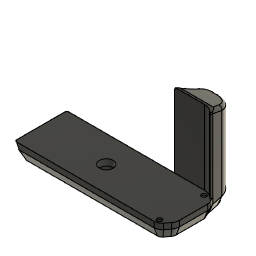
Fujifilm_XE4_Grip (Autodesk Fusion 360 design; units mm, degrees)
Autodesk Fusion 360 part; units mm, degrees
note: some values were not read from the file. Chosen so that the rebuilt part matches the saved one: which pieces of a blend or face edit are solid. Set by a fixed rule: which sketch regions a step uses.
sketch "Boceto1" plane through (0, 0, 0) normal (0, 0, 1) x (1, 0, 0)
  line L0 (-61.186123, 0) -> (71.866078, 0)
  line L1 (-61.186123, 16.5) -> (58.439032, 16.5)
  line L2 (-61.186123, -15.8) -> (59.434444, -15.8)
  line L3 (0, 28.622619) -> (0, -27.140205)
  line L4 (66.8, 10.132205) -> (66.8, -7.372166)
  line L5 (62.761803, 15.128919) -> (63.868179, 14.348585)
  arc A0 (62.761803, 15.128919) -> (58.439032, 16.5) centre (58.439032, 9) ccw
  line L6 (64.040509, 14.215674) -> (65.452845, 13.026924)
  arc A1 (66.8, 10.132205) -> (65.452845, 13.026924) centre (63.016387, 10.132205) ccw
  arc A2 (64.040509, 14.215674) -> (63.868179, 14.348585) centre (62.398436, 12.264752) ccw
  circle A3 centre (52.520822, 19.704936) radius 11.20941
  line L7 (52.520822, 30.914346) -> (49.214141, 30.914346)
  arc A4 (39.279231, 16.5) -> (43.791824, 26.33548) centre (23.188368, 29.835558) ccw
  arc A5 (49.214141, 30.914346) -> (43.791824, 26.33548) centre (49.214141, 25.414346) ccw
  line L8 (41.763113, 20.257885) -> (39.82544, 16.5)
  line L9 (65.452845, 13.026924) -> (63.472116, 22.096594)
  circle A6 centre (62.754834, 14.530444) radius 2.315092
  circle A7 centre (14, 0) radius 4.25
  circle A8 centre (14, 0) radius 6.75
  line L10 (-27, 16.5) -> (-27, -15.8)
  line L11 (35.876287, -15.8) -> (35.876287, -16.8)
  line L12 (35.876287, -16.8) -> (57.161819, -16.8)
  line L13 (57.161819, -16.8) -> (57.161819, -15.8)
  circle A9 centre (60.249431, -13.250185) radius 1.5
  circle A10 centre (60.988338, 13.604964) radius 1.5
  line L14 (63.404093, -13.840047) -> (65.563579, -11.020223)
  arc A11 (59.434444, -15.8) -> (63.404093, -13.840047) centre (59.434444, -10.8) ccw
  arc A12 (65.563579, -11.020223) -> (66.8, -7.372166) centre (60.8, -7.372166) ccw
  dimension "d4" = 7.5
  dimension "d6" = 2.55
  dimension "d7" = 5.5
  dimension "d8" = 8.5
  dimension "d9" = 13.5
  dimension "d14" = 1
  dimension "d15" = 3
  dimension "d16" = 3
  dimension "d17" = 5
  dimension "d18" = 6
  dimension "d41" = 16.5
  dimension "d42" = 15.8
  dimension "d43" = 66.8
  dimension "d44" = 14
  constraint horizontal L0
  constraint perpendicular L2 L3
  constraint parallel L0 L1
  constraint tangent L1 A0
  constraint tangent L5 A0
  constraint parallel L3 L4
  constraint tangent L6 A1
  constraint tangent L4 A1
  constraint tangent L5 A2
  constraint tangent L6 A2
  constraint tangent A3 L7
  constraint horizontal L7
  constraint tangent L7 A5
  constraint tangent A4 A5
  constraint tangent A4 L8
  constraint tangent A3 L9
  constraint tangent L9 A6
  constraint concentric A7 A8
  constraint parallel L0 L2
  constraint perpendicular L2 L11
  constraint perpendicular L11 L12
  constraint perpendicular L2 L13
  constraint tangent L2 A11
  constraint tangent L14 A11
  constraint tangent L14 A12
  constraint tangent L4 A12
  constraint coincident origin L0
  constraint horizontal origin A7.centre
  constraint coincident L1 L10.start
  constraint coincident L2 L10.end
  measures "d4" radius of A0
  measures "d6" radius of A2
  measures "d7" radius of A5
  measures "d8" diameter of A7
  measures "d9" diameter of A8
  measures "d15" diameter of A9
  measures "d16" diameter of A10
  measures "d17" radius of A11
  measures "d18" radius of A12
  measures "d41" distance of L0 L1
  measures "d42" distance of L0 L2
  measures "d43" distance of origin L4
  measures "d44" horizontal distance of origin A7.centre
extrude "Extruir1" add sketch "Boceto1" against normal blind 9 contours L0 A7 A8 | L0 A7 A8 | L0 L1 L3 L4 L6 A1 A3 A6 A8 A10 | L0 L2 L3 L4 A8 L14 A11 A12 | L0 L2 L3 L10 | L0 L1 L3 L10 | L5 A0 L6 A2 A3 A6 A10 | L5 A0 L6 A2 A3 A6 | A3 L9 A6 | A3 A6 A10 | A3 A6 A10 | L1 A0 A3 A4 A5 L8 A6 | A0 A3 A6 | L1 A3 L8 | A3 A6 A10 | A3 A6 A10 | L1 A0 A3 A6 A10 | A3 L7 A5 | A0 A3 A6 A10 | A9 picked at (11.344649, 5.269892) picked at (8.108464, -0.335345) picked at (18.260416, 13.193588) picked at (41.142096, -5.266667) picked at (-18, -5.266667) picked at (-18, 11) picked at (63.509623, 13.402236) picked at (63.825041, 15.302467) picked at (63.810413, 17.600151) picked at (61.317784, 12.424239) picked at (62.039166, 13.392483) picked at (50.353547, 23.728105) picked at (62.520167, 15.99099) picked at (41.048535, 16.816247) picked at (61.414822, 14.237939) picked at (60.789556, 12.505385) picked at (58.292127, 13.195865) picked at (47.006875, 29.774605) picked at (61.192246, 15.569708) picked at (59.87732, -12.98462)
extrude "Extruir2" cut sketch "Boceto1" along normal blind -4 and the other way blind 9 contours L0 A7 A8 | L0 A7 A8 picked at (11.344649, 5.269892) picked at (8.108464, -0.335345)
extrude "Extruir3" add sketch "Boceto1" along normal blind 48 contours L5 A0 L6 A2 A3 A6 | A3 L9 A6 | L1 A0 A3 A4 A5 L8 A6 | A0 A3 A6 | L1 A3 L8 | A3 L7 A5 picked at (63.825041, 15.302467) picked at (63.810413, 17.600151) picked at (50.353547, 23.728105) picked at (62.520167, 15.99099) picked at (41.048535, 16.816247) picked at (47.006875, 29.774605)
sketch "Boceto2" plane through (0, 0, 0) normal (1, 0, 0) x (0, 1, 0)
  line L0 (0, 0) -> (0, 41.347667)
  line L1 (0, 41.347667) -> (34.217677, 41.347667)
  line L2 (31.646617, 41.347667) -> (6.75876, 49.907463)
  line L3 (6.75876, 49.907463) -> (34.217677, 49.907463)
  line L4 (34.217677, 49.907463) -> (34.217677, 41.347667)
  dimension "d45" = 41.347667
  constraint coincident L0.start origin
  constraint vertical L0
  constraint perpendicular L0 L1
  constraint parallel L1 L3
  constraint perpendicular L1 L4
extrude "Extruir4" cut sketch "Boceto2" along normal blind 110 contours L1 L2 L3 L4 picked at (24.207685, 47.054198)
fillet "Empalme1" radius 2 7 edges at (40.794276, 18.378943, 45.91088) (43.011767, 23.218473, 44.246398) (45.665636, 29.616502, 42.045894) (50.867481, 30.914346, 41.59952) (59.550822, 28.435914, 42.451939) (64.244366, 18.560495, 45.848438) (65.054866, 14.266815, 47.325183)
chamfer "Chaflán1" distance 4.2 distance2 9 1 edges at (-27, 0.35, -9) measured on face at (-15.583333, 0.233333, -9)
fillet "Empalme2" radius 9 1 edges at (64.846194, 13.537537, -4.5)
chamfer "Chaflán2" distance 2.2 distance2 5.5 14 edges at (8.51272, 16.5, -9) (43.011767, 23.218473, -9) (40.794276, 18.378943, -9) (18.317222, -15.8, -9) (61.648011, -15.283316, -9) (64.483836, -12.430135, -9) (66.482494, -9.298111, -9) (66.8, 1.38002, -9) (66.648742, 11.19132, -9) (65.47665, 13.571068, -9) (64.238004, 18.589627, -9) (59.550822, 28.435914, -9) (50.867481, 30.914346, -9) (45.665636, 29.616502, -9) measured on face at (-12.783893, 0.233333, -9) measured on face at (-12.783893, 0.233333, -9) measured on face at (-12.783893, 0.233333, -9) measured on face at (-12.783893, 0.233333, -9) measured on face at (-12.783893, 0.233333, -9) measured on face at (-12.783893, 0.233333, -9) measured on face at (-12.783893, 0.233333, -9) measured on face at (-12.783893, 0.233333, -9) measured on face at (-12.783893, 0.233333, -9) measured on face at (65.411059, 13.734607, -6) measured on face at (-12.783893, 0.233333, -9) measured on face at (-12.783893, 0.233333, -9) measured on face at (-12.783893, 0.233333, -9) measured on face at (-12.783893, 0.233333, -9)
chamfer "Chaflán3" distance 0.5 distance2 1 1 edges at (7.70679, -2.440904, -9) measured on face at (-12.783893, 0.233333, -9)
extrude "Extruir5" cut sketch "Boceto1" against normal blind 1 contours A3 A6 A10 | A3 A6 A10 | A3 A6 A10 | A3 A6 A10 | A9 picked at (61.317784, 12.424239) picked at (62.039166, 13.392483) picked at (61.414822, 14.237939) picked at (60.789556, 12.505385) picked at (59.87732, -12.98462)
fillet "Fillet3" radius 1 4 edges at (-24.083333, -14.7, -6.25) (-26.183333, -15.8, -1.75) (-26.183333, 16.5, -1.75) (-24.083333, 15.4, -6.25)
sketch "Trim" plane through (0, 0, 0) normal (0, 1, 0) x (1, 0, 0)
  line L0 (68.315111, -54.700248) -> (37.362685, -54.700248)
  line L1 (37.362685, -54.700248) -> (37.362685, -46.105812)
  line L2 (37.362685, -46.105812) -> (68.315111, -46.105812)
  line L3 (68.315111, -46.105812) -> (68.315111, -54.700248)
  constraint horizontal L0
  constraint vertical L1
  constraint horizontal L2
  constraint vertical L3
extrude "Extrude6" cut sketch "Trim" along normal blind 29 contours L0 L1 L2 L3 picked at (47.68016, -51.835436)
named bodies: "Grip"
